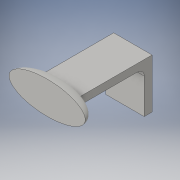
# Autodesk Inventor part: Camera
Saved by Autodesk Inventor 2016 (Build 200138000, 138)
## iProperties
Created: 2015-09-18
Part Number: Camera
Material: Generic
Document SubType Name: Modeling
Designer: lachesis
Density: 1 g/cm^3
Appearance: Default
Author: lachesis
Autodesk Inventor part; units mm, degrees
ref_plane "YZ Plane" through (0, 0, 0) normal (1, 0, 0) x (0, 1, 0)
ref_plane "XZ Plane" through (0, 0, 0) normal (0, 1, 0) x (-1, 0, 0)
ref_plane "XY Plane" through (0, 0, 0) normal (0, 0, 1) x (1, 0, 0)
sketch "Sketch1" plane through (0, 0, 0) normal (0, 0, 1) x (1, 0, 0)
  ellipse E0 centre (0, 0) end of major axis (35.052, 0) minor radius 14.859 (35.052, 0) -> (-35.052, 0) ccw
  line L0 (35.052, 0) -> (-35.052, 0)
  dimension "d0" = 14.859
  dimension "d1" = 35.052
  constraints: 2 end point, 1 coincident, 1 horizontal, 1 horizontal alignment, 4 other
revolve "Revolution1" add sketch "Sketch1" angle 180 about axis through (35.052, 0, 0) along (-1, 0, 0)
ref_plane "Work Plane1" through (0, 0, -10.16) normal (0, 0, 1) x (1, 0, 0)
sketch "Sketch2" plane through (0, 0, -10.16) normal (0, 0, 1) x (1, 0, 0)
  line L0 (17.653, 3.429) -> (-17.653, 3.429)
  line L1 (-17.653, 3.429) -> (-17.653, -3.429)
  line L2 (-17.653, -3.429) -> (17.653, -3.429)
  line L3 (17.653, -3.429) -> (17.653, 3.429)
  point P0 (0, 0)
  point P1 (0, 3.429)
  point P2 (17.653, 0)
  dimension "d4" = 35.306
  dimension "d5" = 6.858
  constraints: 8 end point, 2 midpoint, 2 parallel, 1 horizontal, 1 horizontal alignment, 1 perpendicular, 1 vertical alignment
  measures "d4" distance of L0.start L0.end
  measures "d5" distance of L0.end L1.end
extrude "Extrusion1" add sketch "Sketch2" against normal blind 68.707
sketch "Sketch3" plane through (0, 0, -78.867) normal (0, 0, -1) x (-1, 0, 0)
  line L0 (17.653, 3.429) -> (-17.653, 3.429) projected
  line L1 (-17.653, 3.429) -> (-17.653, -3.429) projected
  line L2 (-17.653, -3.429) -> (17.653, -3.429) projected
  line L3 (17.653, -3.429) -> (17.653, 3.429) projected
  line L4 (17.653, 3.429) -> (-17.653, 3.429) projected
  line L5 (-17.653, 3.429) -> (17.653, 3.429)
  line L6 (17.653, 3.429) -> (17.653, -42.037)
  line L7 (17.653, -42.037) -> (-17.653, -42.037)
  line L8 (-17.653, -42.037) -> (-17.653, 3.429)
  point P0 (0, 0)
  dimension "d8" = 45.466
  constraints: 8 end point, 2 parallel, 1 horizontal, 1 perpendicular
  measures "d8" distance of L0.start L6.end
extrude "Extrusion2" add sketch "Sketch3" against normal blind 7.239 contours L6 L7 L8 L2
sketch "Sketch4" plane through (-17.653, -3.429, -71.628) normal (0, -1, 0) x (1, 0, 0)
  line L0 (27.559, 49.784) -> (7.747, 49.784)
  line L1 (7.747, 49.784) -> (7.747, 47.244)
  line L2 (7.747, 47.244) -> (27.559, 47.244)
  line L3 (27.559, 47.244) -> (27.559, 49.784)
  line L4 (0, 0) -> (35.306, 0) projected
  point P0 (17.653, 71.628)
  point P1 (17.653, 47.244)
  point P2 (17.653, 0)
  dimension "d11" = 47.244
  dimension "d12" = 2.54
  dimension "d13" = 19.812
  constraints: 8 end point, 2 midpoint, 2 parallel, 1 horizontal, 1 perpendicular, 1 vertical alignment
  measures "d11" distance between parallel lines of L2 L4
  measures "d12" distance of L0.end L1.end
  measures "d13" distance of L0.start L0.end
extrude "Extrusion3" add sketch "Sketch4" along normal blind 9.906
fillet "Fillet1" radius 6.35 1 edges at (0, -3.429, -71.628)
fillet "Fillet2" radius 1.27 1 edges at (0, -3.429, -24.384)
body "Solid1"
